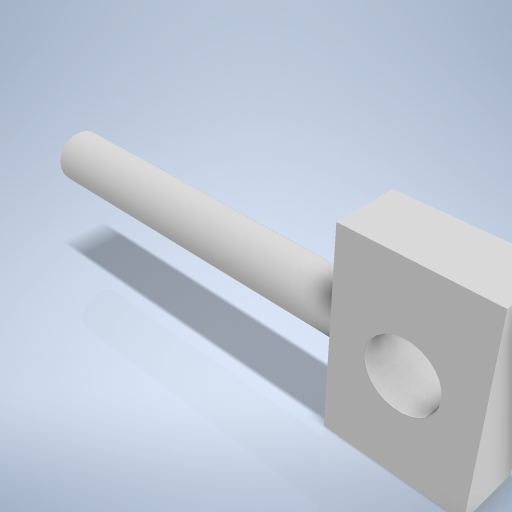
# Autodesk Inventor part: pleuel_m4
Saved by Autodesk Inventor 2024.2 (Build 282272000, 272)
## iProperties
Created: 2024-05-15
Part Number: pleuel_m4
Material: Generisch
Document SubType Name: Modeling
Designer: Fabri
Density: 1 g/cm^3
Appearance: Vorgabe
Author: Fabri
Autodesk Inventor part; units mm, degrees
ref_plane "YZ Plane" through (0, 0, 0) normal (1, 0, 0) x (0, 1, 0)
ref_plane "XZ Plane" through (0, 0, 0) normal (0, 1, 0) x (-1, 0, 0)
ref_plane "XY Plane" through (0, 0, 0) normal (0, 0, 1) x (1, 0, 0)
sketch "Skizze2" plane through (0, 0, 0) normal (0, 1, 0) x (-1, 0, 0)
  line L0 (-6.5, 9.5) -> (6.5, 9.5)
  line L1 (6.5, 9.5) -> (6.5, -9.5)
  line L2 (6.5, -9.5) -> (-6.5, -9.5)
  line L3 (-6.5, -9.5) -> (-6.5, 9.5)
  line L4 (-6.5, 9.5) -> (6.5, -9.5) construction
  line L5 (6.5, 9.5) -> (-6.5, -9.5) construction
  point P0 (0, 0)
  dimension "d1" = 19
  dimension "d2" = 13
  constraints: 12 end point, 2 midpoint, 2 parallel, 1 horizontal, 1 perpendicular
  measures "d1" distance between parallel lines of L2 L0
  measures "d2" distance between parallel lines of L3 L1
extrude "Extrusion1" add sketch "Skizze2" along normal blind 6
sketch "Skizze3" plane through (0, 6, 0) normal (0, 1, 0) x (1, 0, 0)
  point P0 (0, 0)
  point P1 (0, 0)
  constraints: 1 coincident
hole "Bohrung1" at (0, 6, 0) direction (0, -1, 0) diameter 6.5 depth 6
sketch "Skizze4" plane through (-6.5, 0, -9.5) normal (-1, 0, 0) x (0, 0, 1)
  circle A0 centre (9.5, 3) radius 2.5
  line L0 (0, 0) -> (0, 6) projected
  line L1 (0, 0) -> (19, 0) projected
  point P0 (9.5, 0)
  point P1 (0, 3)
  point P2 (9.5, 0)
  dimension "d12" = 5
  constraints: 2 midpoint, 1 centre point, 1 horizontal alignment, 1 vertical alignment
  measures "d12" diameter of A0
extrude "Extrusion2" add sketch "Skizze4" along normal blind 34
sketch "Skizze5" plane through (-40.5, 3, 0) normal (-1, 0, 0) x (0, 0, 1)
  circle A0 centre (0, 0) radius 2.5 projected
  point P0 (0, -3)
  constraints: 1 coincident
hole "Bohrung2" at (-40.5, 3, 0) direction (1, 0, 0) diameter 3.242 depth 5 thread size "M4x0.7" class "6H" standard "ISO Metric profile"
